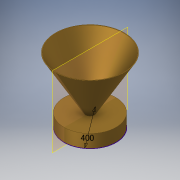
# Autodesk Inventor part: thruster
Saved by Autodesk Inventor 2019.1 (Build 231200000, 200)
## iProperties
Created: 2018-12-21
Part Number: thruster
Material: 真鍮、ソフト イエロー
Document SubType Name: Modeling
Designer: Masaya
Density: 8.47 g/cm^3
Appearance: 真鍮 - サテン
Author: Masaya
Autodesk Inventor part; units mm, degrees
ref_plane "XZ Plane" through (0, 0, 0) normal (0, 1, 0) x (-1, 0, 0)
ref_plane "XY Plane" through (0, 0, 0) normal (0, 0, 1) x (1, 0, 0)
sketch "スケッチ1" plane through (0, 0, 0) normal (0, 1, 0) x (-1, 0, 0)
  circle A0 centre (0, 0) radius 200
  dimension "d0" = 400
  constraints: 1 centre point, 1 coincident
  measures "d0" diameter of A0
extrude "押し出し1" add sketch "スケッチ1" along normal blind 100
sketch "スケッチ2" plane through (0, 0, 0) normal (1, 0, 0) x (0, 1, 0)
  line L0 (100, -200) -> (100, 200) projected
  line L1 (0, 200) -> (0, -200) projected
  line L2 (100, -200) -> (100, 200) projected
  line L3 (100, 35) -> (500, 265.9401)
  line L4 (500, 265.9401) -> (500, 260.9401)
  line L5 (500, 260.9401) -> (100, 30)
  line L6 (100, 35) -> (100, 30)
  line L7 (-70, 0) -> (420, 0) projected
  point P0 (0, 0)
  point P1 (100, 0)
  dimension "d3" = 5
  dimension "d4" = 5
  dimension "d5" = 400
  dimension "d6" = 60
  dimension "d7" = 35
  constraints: 8 end point, 2 point on line, 1 collinear, 1 midpoint, 1 parallel
  measures "d3" distance of L3.end L4.end
  measures "d4" distance of L5.end L3.start
  measures "d5" distance from line of L0 L3.end
  measures "d6" angle of L0 L3
  measures "d7" distance of L3.start point (100, 0)
revolve "回転1" add sketch "スケッチ2" angle 360 about axis through (0, -10, 0) along (0, 1, 0)
